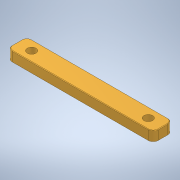
# Autodesk Inventor part: Lower Arm Brass Plate - 3
Saved by Autodesk Inventor 2021.1 (Build 251245010, 245A)
## iProperties
Created: 2025-09-16
Material: Brass, Soft Yellow
Document SubType Name: Modeling
Designer: SD
Density: 8.47 g/cm^3
Appearance: Brass - Satin
Mass: 243.323 g
Surface Area: 97.1102 cm^2
Volume: 28.7277 cm^3
Project: Automatic Tea Steeping mechanism
Part Number: Lower Arm Brass Plate - 3
Length: 150.000 mm
Width: 20.000 mm
Thickness: 10.000 mm
BOM-Mass: 0.24332
BOM-Area: 0.010
Author: SD
Title: Lower Arm Brass Plate - 3
Autodesk Inventor part; units mm, degrees
ref_plane "YZ Plane" through (0, 0, 0) normal (1, 0, 0) x (0, 1, 0)
ref_plane "XZ Plane" through (0, 0, 0) normal (0, 1, 0) x (-1, 0, 0)
ref_plane "XY Plane" through (0, 0, 0) normal (0, 0, 1) x (1, 0, 0)
sketch "Sketch1" plane through (0, 0, 0) normal (0, 1, 0) x (-1, 0, 0)
  line L0 (-75, 10) -> (75, 10)
  line L1 (75, 10) -> (75, -10)
  line L2 (75, -10) -> (-75, -10)
  line L3 (-75, -10) -> (-75, 10)
  line L4 (-75, 10) -> (75, -10) construction
  line L5 (75, 10) -> (-75, -10) construction
  point P0 (0, 0)
  dimension "Length" = 150
  dimension "Width" = 20
  constraints: 12 end point, 2 midpoint, 2 parallel, 1 horizontal, 1 perpendicular
  measures "Length" distance of L1.end L2.end
  measures "Width" distance of L0.end L1.end
extrude "Extrusion1" add sketch "Sketch1" along normal mid plane 10
sketch "Sketch4" plane through (0, 5, 0) normal (0, 1, 0) x (1, 0, 0)
  point P0 (0, 0)
  point P1 (-60, 0)
  point P2 (60, 0)
  dimension "d16" = 120
  dimension "d17" = 60
  constraints: 2 horizontal alignment
  measures "d16" distance of point (60, 0) point (-60, 0)
  measures "d17" distance of point (0, 0) point (60, 0)
hole "Hole2" at (-60, 5, 0) at (60, 5, 0) direction (0, -1, 0) diameter 9 end through all
fillet "Fillet1" radius 5 4 edges at (75, 0, 10) (75, 0, -10) (-75, 0, 10) (-75, 0, -10)
chamfer "Chamfer2" distance 0.5 angle 45 8 edges at (0, 5, 10) (73.5355, 5, 8.5355) (75, 5, 0) (73.5355, 5, -8.5355) (0, 5, -10) (-73.5355, 5, -8.5355) (-75, 5, 0) (-73.5355, 5, 8.5355)
equation "\"d17\" = 0.5 * d16"
body "Solid1"
